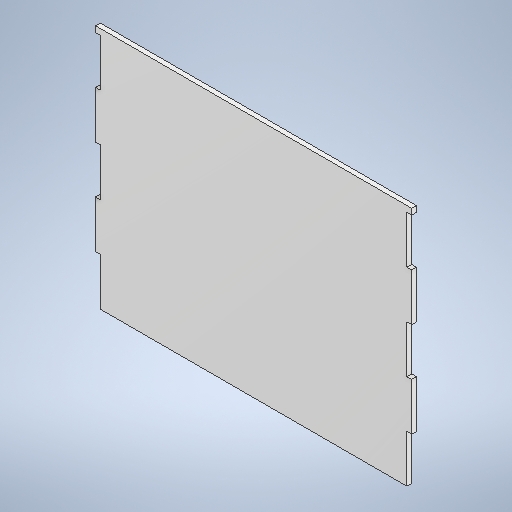
# Autodesk Inventor part: Q side 3
Saved by Autodesk Inventor 2025.3 (Build 293356000, 356)
## iProperties
Created: 2026-04-17
Part Number: Q side 3
Material: ABS Plastic
Document SubType Name: Modeling
Designer: logien
Density: 1.06 g/cm^3
Appearance: Smooth - White
Author: logien
Autodesk Inventor part; units mm, degrees
ref_plane "YZ Plane" through (0, 0, 0) normal (1, 0, 0) x (0, 1, 0)
ref_plane "XZ Plane" through (0, 0, 0) normal (0, 1, 0) x (-1, 0, 0)
ref_plane "XY Plane" through (0, 0, 0) normal (0, 0, 1) x (1, 0, 0)
sketch "Sketch1" plane through (0, 0, 0) normal (0, 0, 1) x (1, 0, 0)
  line L0 (0, 0) -> (200, 0)
  line L1 (0, 0) -> (3, 0)
  line L2 (3, 0) -> (3, 30)
  line L3 (3, 30) -> (0, 30)
  line L4 (0, 30) -> (0, 60)
  line L5 (0, 60) -> (3, 60)
  line L6 (3, 60) -> (3, 90)
  line L7 (3, 90) -> (0, 90)
  line L8 (0, 90) -> (0, 120)
  line L9 (0, 120) -> (3, 120)
  line L10 (3, 120) -> (3, 150)
  line L11 (3, 150) -> (0, 150)
  line L12 (0, 150) -> (0, 153.75)
  line L13 (100, 153.75) -> (100, 0)
  line L14 (200, 0) -> (197, 0)
  line L15 (197, 0) -> (197, 30)
  line L16 (197, 30) -> (200, 30)
  line L17 (200, 30) -> (200, 60)
  line L18 (200, 60) -> (197, 60)
  line L19 (197, 60) -> (197, 90)
  line L20 (197, 90) -> (200, 90)
  line L21 (200, 90) -> (200, 120)
  line L22 (200, 120) -> (197, 120)
  line L23 (197, 120) -> (197, 150)
  line L24 (197, 150) -> (200, 150)
  line L25 (200, 150) -> (200, 153.75)
  line L26 (0, 150) -> (0, 153.75)
  line L27 (0, 153.75) -> (200, 153.75)
  dimension "d0" = 200
  dimension "d2" = 3
  dimension "d3" = 30
  dimension "d4" = 3
  dimension "d5" = 30
  dimension "d6" = 3
  dimension "d7" = 30
  dimension "d8" = 3
  dimension "d9" = 30
  dimension "d10" = 3
  dimension "d11" = 30
  dimension "d12" = 3
  dimension "d16" = 3.75
  constraints: 56 end point, 11 symmetric about line, 9 point on line, 5 parallel, 2 midpoint, 1 horizontal, 1 perpendicular
  measures "d0" distance of L0.start L0.end
  measures "d2" distance of L0.start L1.end
  measures "d3" distance of L1.end L2.end
  measures "d4" distance of L2.end L3.end
  measures "d5" distance of L3.end L4.end
  measures "d6" distance of L4.end L5.end
  measures "d7" distance of L5.end L6.end
  measures "d8" distance of L6.end L7.end
  measures "d9" distance of L7.end L8.end
  measures "d10" distance of L8.end L9.end
  measures "d11" distance of L9.end L10.end
  measures "d12" distance of L10.end L11.end
  measures "d16" distance of L12.end L11.end
extrude "Extrusion1" add sketch "Sketch1" along normal blind 3
body "Solid1"
